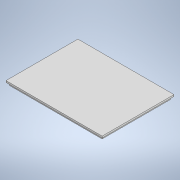
# Autodesk Inventor part: cap
Saved by Autodesk Inventor 2021 (Build 250183000, 183)
## iProperties
Created: 2020-11-03
Part Number: cap
Material: Generic
Document SubType Name: Modeling
Designer: s094623
Density: 1 g/cm^3
Appearance: Default
Author: s094623
Autodesk Inventor part; units mm, degrees
ref_plane "YZ Plane" through (0, 0, 0) normal (1, 0, 0) x (0, 1, 0)
ref_plane "XZ Plane" through (0, 0, 0) normal (0, 1, 0) x (-1, 0, 0)
ref_plane "XY Plane" through (0, 0, 0) normal (0, 0, 1) x (1, 0, 0)
sketch "Sketch1" plane through (0, 0, 0) normal (0, 1, 0) x (-1, 0, 0)
  line L0 (0, 0) -> (0, 86)
  line L1 (0, 86) -> (-115, 86)
  line L2 (-115, 86) -> (-115, 0)
  line L3 (-115, 0) -> (0, 0)
  dimension "d0" = 86
  dimension "d1" = 115
  constraints: 8 end point, 3 perpendicular, 1 vertical
  measures "d0" distance of L0.start L0.end
  measures "d1" distance of L0.end L1.end
extrude "Extrusion1" add sketch "Sketch1" along normal blind 2
sketch "Sketch2" plane through (0, 0, 0) normal (0, -1, 0) x (1, 0, 0)
  point P0 (0, 0)
sketch "Sketch3" plane through (0, 0, 0) normal (0, -1, 0) x (1, 0, 0)
  line L0 (112, 83) -> (3, 83)
  line L1 (3, 83) -> (3, 3)
  line L2 (3, 3) -> (112, 3)
  line L3 (112, 3) -> (112, 83)
  line L4 (4, 82) -> (111, 82)
  line L5 (111, 82) -> (111, 4)
  line L6 (111, 4) -> (4, 4)
  line L7 (4, 4) -> (4, 82)
  point P0 (0, 0)
  dimension "d4" = 109
  dimension "d5" = 80
  dimension "d6" = 109
  dimension "d7" = 1
  constraints: 16 end point, 2 perpendicular, 1 horizontal, 1 vertical, 3 other
  measures "d4" distance of L0.start L0.end
  measures "d5" distance of L0.end L1.end
  measures "d6" distance of L1.end L2.end
  measures "d7" distance between parallel lines of L0 L4
extrude "Extrusion2" add sketch "Sketch3" along normal blind 3
sketch "Sketch4" plane through (0, -3, 0) normal (0, -1, 0) x (1, 0, 0)
  line L0 (2, 84) -> (113, 84)
  line L1 (113, 84) -> (113, 2)
  line L2 (113, 84) -> (195, 84) construction
  line L3 (113, 2) -> (2, 2)
  line L4 (3, 3) -> (112, 3) projected
  line L5 (2, 2) -> (2, 84)
  line L6 (112, 3) -> (112, 83)
  line L7 (112, 83) -> (3, 83)
  line L8 (3, 83) -> (3, 3)
  line L9 (3, 3) -> (112, 3)
  point P0 (0, 0)
  dimension "d10" = 111
  dimension "d11" = 82
  dimension "d12" = 90
  dimension "d13" = 111
  dimension "d14" = 90
  constraints: 18 end point, 2 horizontal, 1 parallel, 1 perpendicular, 1 vertical, 3 other
  measures "d10" distance of L0.start L0.end
  measures "d11" distance of L0.end L1.end
  measures "d12" angle of L1 L2
  measures "d13" distance of L1.end L3.end
  measures "d14" angle of L1 L3
extrude "Extrusion3" add sketch "Sketch4" against normal blind 1
body "Solid1"
